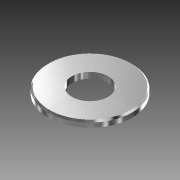
# Autodesk Inventor part: arandela m3
Saved by Autodesk Inventor 2012 SP2 (Build 160219200, 219)
## iProperties
Shininess: 64.0
Length Units: 11269
Angle Units: 11279
Time Units: 11290
Mass Units: 11283
Length Display Precision: 3
Angle Display Precision: 2
Compacted: True
Created: 2002-08-23
Part Number: arandela m3
Material: 140 HV
Description: DIN 125-B / ISO 7090 - M18
Document SubType Name: Modeling
Designer: Cor de Vlaming
Density: 7.84 g/cm^3
Density: 0.0
Volumn: 0.0
Area: 0.0
PropertySet Name: Model Information
Control State: 0
Master: False
Checked Out: False
Author: Cor de Vlaming
Autodesk Inventor part; units mm, degrees
ref_plane "YZ Plane" through (0, 0, 0) normal (1, 0, 0) x (0, 1, 0)
ref_plane "XZ Plane" through (0, 0, 0) normal (0, 1, 0) x (-1, 0, 0)
ref_plane "XY Plane" through (0, 0, 0) normal (0, 0, 1) x (1, 0, 0)
sketch "Sketch3" plane through (0, 0, 0) normal (0, 0, 1) x (1, 0, 0)
  circle A0 centre (0, 0) radius 1.5
  circle A1 centre (0, 0) radius 3.5
  dimension "d1" = 3
  dimension "d2" = 7
  constraints: 2 centre point, 1 coincident
  measures "d1" diameter of A0
  measures "d2" diameter of A1
extrude "Extrusion2" add sketch "Sketch3" along normal blind 0.5
chamfer "Chamfer2" distance 0.125 angle 45 1 edges at (-3.5, 0, 0.5)
equation "\"d8\" = 0.25 * h"
equation "\"d9\" = 0.25 * h"
equation "\"h\" = 0.5"
